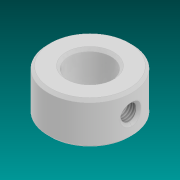
# Autodesk Inventor part: stelring - 8mm
Saved by Autodesk Inventor 2020 (Build 240168000, 168)
## iProperties
Created: 2020-05-17
Part Number: stelring - 8mm
Material: Generic
Document SubType Name: Modeling
Designer: stefa
Density: 1 g/cm^3
Appearance: Default
Author: stefa
Autodesk Inventor part; units mm, degrees
ref_plane "XZ Plane" through (0, 0, 0) normal (0, 1, 0) x (-1, 0, 0)
ref_plane "XY Plane" through (0, 0, 0) normal (0, 0, 1) x (1, 0, 0)
sketch "Sketch1" plane through (0, 0, 0) normal (0, 1, 0) x (-1, 0, 0)
  circle A0 centre (0, 0) radius 4
  circle A1 centre (0, 0) radius 7.95
  dimension "d0" = 8
  dimension "d1" = 15.9
  constraints: 2 centre point, 2 coincident
  measures "d0" diameter of A0
  measures "d1" diameter of A1
extrude "Extrusion1" add sketch "Sketch1" along normal blind 8
ref_plane "Work Plane1" through (7.95, 0, 0) normal (1, 0, 0) x (0, 1, 0)
sketch "Sketch2" plane through (7.95, 0, 0) normal (1, 0, 0) x (0, 1, 0)
  circle A0 centre (4, 0) radius 1.5
  line L0 (0, -7.95) -> (0, 7.95) projected
  line L1 (8, -7.95) -> (8, 7.95) projected
  point P0 (0, 0)
  dimension "d4" = 3
  dimension "d5" = 8
  dimension "d6" = 4
  constraints: 1 centre point, 1 horizontal alignment
  measures "d4" diameter of A0
  measures "d5" distance between parallel lines of L0 L1
  measures "d6" distance of point (0, 0) A0.centre
extrude "Extrusion2" cut sketch "Sketch2" against normal up to surface round surface about axis through (0, 0, 0) along (0, 1, 0) radius 4 far side no
thread "Thread1" size "M3x0.5" class "6H" standard "ANSI Metric M Profile" full length
chamfer "Chamfer1" distance 0.5 angle 45 7 edges at (7.95, 8, 0) (4, 8, 0) (7.95, 0, 0) (4, 0, 0) (4, 2.5, 0.0024) (7.8072, 3.9998, -1.5) (7.8072, 4.0001, 1.5)
equation "\"d6\" = 0.5 * d5"
body "Solid1"
